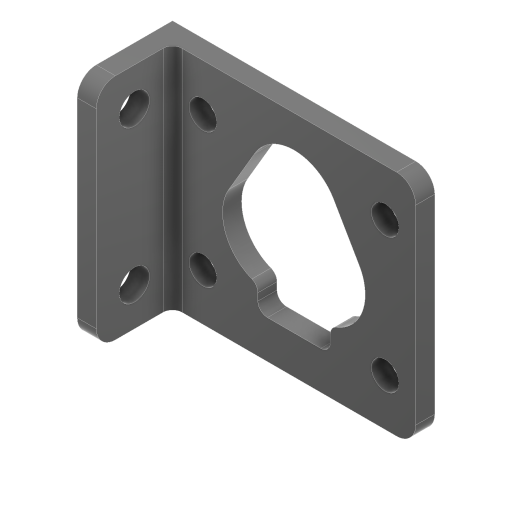
# Autodesk Inventor part: CAN Resistor Mount
Saved by Autodesk Inventor 2023 (Build 270158000, 158)
## iProperties
Created: 2023-12-17
Part Number: CAN Resistor Mount
Material: Generic
Document SubType Name: Modeling
Designer: Adam Arnold
Density: 1 g/cm^3
Appearance: Smooth - Black
Author: Adam Arnold
Autodesk Inventor part; units mm, degrees
ref_plane "YZ Plane" through (0, 0, 0) normal (1, 0, 0) x (0, 1, 0)
ref_plane "XZ Plane" through (0, 0, 0) normal (0, 1, 0) x (-1, 0, 0)
ref_plane "XY Plane" through (0, 0, 0) normal (0, 0, 1) x (1, 0, 0)
sketch "Sketch1" plane through (0, 0, 0) normal (0, 0, 1) x (1, 0, 0)
  line L0 (0, 0) -> (43.688, 0)
  line L1 (43.688, 0) -> (43.688, 38.1)
  line L2 (43.688, 38.1) -> (0, 38.1)
  line L3 (0, 38.1) -> (0, 0)
  dimension "d0" = 43.688
  dimension "d1" = 38.1
  constraints: 8 end point, 2 parallel, 1 horizontal, 1 perpendicular
  measures "d0" distance of L1.end L2.end
  measures "d1" distance of L0.end L1.end
extrude "Extrusion1" add sketch "Sketch1" along normal blind 3.175
sketch "Sketch2" plane through (0, 0, 3.175) normal (0, 0, 1) x (1, 0, 0)
  line L0 (43.688, 38.1) -> (0, 38.1) projected
  line L1 (0, 0) -> (43.688, 0) projected
  line L2 (0, 38.1) -> (3.175, 38.1)
  line L3 (3.175, 38.1) -> (3.175, 0)
  line L4 (3.175, 0) -> (0, 0)
  line L5 (0, 0) -> (0, 38.1)
  dimension "d4" = 3.175
  constraints: 8 end point, 2 parallel, 1 horizontal, 1 perpendicular, 1 point on line
  measures "d4" distance of L3.end L4.end
extrude "Extrusion2" add sketch "Sketch2" along normal blind 12.7
sketch "Sketch4" plane through (0, 0, 3.175) normal (0, 0, 1) x (1, 0, 0)
  line L0 (43.688, 38.1) -> (3.175, 38.1) projected
  line L1 (43.688, 0) -> (43.688, 38.1) projected
  point P0 (0, 0)
  point P1 (38.608, 30.2768)
  point P2 (40.513, 38.1)
  point P3 (6.35, 38.1)
  point P4 (43.688, 3.175)
  point P5 (43.688, 34.925)
  dimension "d8" = 7.8232
  dimension "d9" = 5.08
  measures "d8" distance from line of L0 point (38.608, 30.277)
  measures "d9" distance from line of L1 point (38.608, 30.277)
hole "Hole1" at (38.608, 30.2768, 3.175) direction (0, 0, -1) diameter 4.572 end through all
sketch "Sketch5" plane through (0, 0, 3.175) normal (0, 0, 1) x (1, 0, 0)
  line L0 (3.175, 0) -> (43.688, 0) projected
  line L1 (43.688, 0) -> (43.688, 38.1) projected
  point P0 (0, 0)
  point P1 (38.608, 7.8232)
  point P2 (6.35, 0)
  point P3 (40.513, 0)
  point P4 (43.688, 3.175)
  point P5 (43.688, 34.925)
  dimension "d17" = 7.8232
  dimension "d18" = 5.08
  measures "d17" distance from line of L0 point (38.608, 7.823)
  measures "d18" distance from line of L1 point (38.608, 7.823)
hole "Hole2" at (38.608, 7.8232, 3.175) direction (0, 0, -1) diameter 4.572 end through all
sketch "Sketch6" plane through (3.175, 0, 3.175) normal (1, 0, 0) x (0, 0, -1)
  line L0 (-12.7, 0) -> (-12.7, 38.1) projected
  line L1 (0, 38.1) -> (-12.7, 38.1) projected
  point P0 (3.175, 0)
  point P1 (-6.35, 31.75)
  dimension "d26" = 6.35
  dimension "d27" = 6.35
  measures "d26" distance from line of L0 point (-6.35, 31.75)
  measures "d27" distance from line of L1 point (-6.35, 31.75)
hole "Hole3" at (3.175, 31.75, 9.525) direction (-1, 0, 0) diameter 5.0038 end through all
sketch "Sketch7" plane through (3.175, 0, 3.175) normal (1, 0, 0) x (0, 0, -1)
  line L0 (-12.7, 0) -> (-12.7, 38.1) projected
  line L1 (0, 0) -> (-12.7, 0) projected
  point P0 (3.175, 0)
  point P1 (-6.35, 6.35)
  dimension "d35" = 6.35
  dimension "d36" = 6.35
  measures "d35" distance from line of L0 point (-6.35, 6.35)
  measures "d36" distance from line of L1 point (-6.35, 6.35)
hole "Hole4" at (3.175, 6.35, 9.525) direction (-1, 0, 0) diameter 5.0038 end through all
fillet "Fillet3" radius 3.175 4 edges at (1.5875, 38.1, 15.875) (1.5875, 0, 15.875) (43.688, 38.1, 1.5875) (43.688, 0, 1.5875)
fillet "Fillet4" radius 1.5875 1 edges at (3.175, 19.05, 3.175)
sketch "Sketch8" plane through (0, 0, 3.175) normal (0, 0, 1) x (1, 0, 0)
  line L0 (43.688, 3.175) -> (43.688, 34.925) projected
  line L1 (40.513, 38.1) -> (4.7625, 38.1) projected
  point P0 (0, 0)
  point P1 (8.2296, 30.2768)
  dimension "d47" = 35.4584
  dimension "d48" = 7.8232
  measures "d47" distance from line of L0 point (8.23, 30.277)
  measures "d48" distance from line of L1 point (8.23, 30.277)
hole "Hole5" at (8.2296, 30.2768, 3.175) direction (0, 0, -1) diameter 4.572 end through all
sketch "Sketch9" plane through (0, 0, 3.175) normal (0, 0, 1) x (1, 0, 0)
  line L0 (4.7625, 0) -> (40.513, 0) projected
  line L1 (43.688, 3.175) -> (43.688, 34.925) projected
  point P0 (0, 0)
  point P1 (8.2296, 7.8232)
  dimension "d56" = 7.8232
  dimension "d57" = 35.4584
  measures "d56" distance from line of L0 point (8.23, 7.823)
  measures "d57" distance from line of L1 point (8.23, 7.823)
hole "Hole6" at (8.2296, 7.8232, 3.175) direction (0, 0, -1) diameter 4.572 end through all
sketch "Sketch10" plane through (0, 0, 3.175) normal (0, 0, 1) x (1, 0, 0)
  line L0 (19.2024, 17.78) -> (27.6606, 17.78) construction
  line L1 (23.4315, 17.78) -> (23.4315, 25.1206) construction
  line L2 (43.688, 3.175) -> (43.688, 34.925) projected
  line L3 (4.7625, 0) -> (40.513, 0) projected
  line L4 (19.2024, 11.43) -> (27.6606, 11.43)
  line L5 (28.9337, 28.2905) -> (33.1628, 20.9499)
  arc A0 (29.6452, 23.8119) -> (23.4315, 13.0432) centre (27.6606, 17.78) ccw construction
  arc A1 (27.6606, 11.43) -> (33.1628, 20.9499) centre (27.6606, 17.78) ccw
  line L6 (17.9293, 28.2905) -> (13.7002, 20.9499)
  arc A2 (23.4315, 13.0432) -> (17.2178, 23.8119) centre (19.2024, 17.78) ccw construction
  arc A3 (13.7002, 20.9499) -> (19.2024, 11.43) centre (19.2024, 17.78) ccw
  arc A4 (28.9337, 28.2905) -> (17.9293, 28.2905) centre (23.4315, 25.1206) ccw
  arc A5 (17.2178, 23.8119) -> (29.6452, 23.8119) centre (23.4315, 25.1206) ccw construction
  line L7 (16.8289, 28.9245) -> (12.5407, 21.618)
  arc A6 (12.5407, 21.618) -> (17.399, 10.3063) centre (19.2024, 17.78) ccw
  arc A7 (29.464, 10.3765) -> (34.2632, 21.5839) centre (27.6606, 17.78) ccw
  line L8 (34.2632, 21.5839) -> (30.0341, 28.9245)
  arc A8 (30.0341, 28.9245) -> (16.8289, 28.9245) centre (23.4315, 25.1206) ccw
  line L9 (17.399, 6.35) -> (29.464, 6.35)
  line L10 (23.4315, 6.35) -> (23.4315, 4.7621) construction
  line L11 (17.399, 6.35) -> (17.399, 10.3063)
  line L12 (29.464, 6.35) -> (29.464, 10.3765)
  point P0 (0, 0)
  dimension "d65" = 8.4582
  dimension "d71" = 7.3406
  dimension "d72" = 20.2565
  dimension "d73" = 17.78
  dimension "d74" = 1.27
  dimension "d75" = 11.43
  dimension "d76" = 12.065
  dimension "d77" = 0
  constraints: 22 end point, 18 point on circle, 9 centre point, 6 tangent, 3 vertical, 2 horizontal, 2 midpoint, 1 coincident, 1 horizontal alignment, 1 parallel, 1 perpendicular, 1 other
  measures "d65" distance of L0.end L0.start
  measures "d71" distance of L1.start L1.end
  measures "d72" distance from line of L2 L1.start
  measures "d73" distance from line of L3 L1.start
  measures "d74" radial gap between concentric circles of A4 A8
  measures "d75" distance between parallel lines of L0 L9
  measures "d76" distance of L9.start L9.end
  measures "d77" distance from line of A4.centre L10
extrude "Extrusion3" cut sketch "Sketch10" against normal through all contours A3 L6 A4 L5 A1 L4 | A8 L8 A7 L12 L9 L11 A6 L7
fillet "Fillet5" radius 1.5875 2 edges at (17.399, 6.35, 1.5875) (29.464, 6.35, 1.5875)
fillet "Fillet6" radius 1.5875 2 edges at (17.399, 10.3063, 1.5875) (29.464, 10.3765, 1.5875)
body "Solid1"
